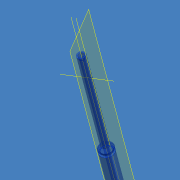
# Autodesk Inventor part: Halter02
Saved by Autodesk Inventor 2013 (Build 170138000, 138)
## iProperties
Created: 2006-08-08
Part Number: Halter02
Document SubType Name: Modeling
Designer: acad
Manufacturer: Standard
Standards Organization: Custom
Material: Allgemein
Density: 1 g/cm^3
Author: acad
Autodesk Inventor part; units mm, degrees
ref_plane "YZ Plane" through (0, 0, 0) normal (1, 0, 0) x (0, 1, 0)
ref_plane "XZ Plane" through (0, 0, 0) normal (0, 1, 0) x (-1, 0, 0)
ref_plane "XY Plane" through (0, 0, 0) normal (0, 0, 1) x (1, 0, 0)
sketch "Skizze1" plane through (0, 0, 0) normal (0, 0, 1) x (1, 0, 0)
  line L0 (-0.0085, 0) -> (-0.0085, 9)
  line L1 (-7.0085, 16) -> (-15.0085, 16)
  line L2 (-15.0085, 16) -> (-15.0085, 7)
  line L3 (-30.0085, 5.925) -> (-111.1085, 5.925)
  line L4 (-113.8085, 5.925) -> (-115.0085, 5.925)
  line L5 (-115.0085, 5.925) -> (-117.4335, 3.5)
  line L6 (-117.4335, 3.5) -> (-204.9135, 3.5)
  line L7 (-204.9135, 3.5) -> (-204.9135, 0)
  line L8 (-222.883, 3.2454) -> (-222.883, 3.2454)
  line L9 (-222.883, 3.2454) -> (-222.883, 3.2454)
  line L10 (-204.9135, 0) -> (-0.0085, 0)
  line L11 (-111.8085, 4.5) -> (-113.1085, 4.5)
  line L12 (-30.0085, 5.925) -> (-29.0085, 7)
  line L13 (-29.0085, 7) -> (-15.0085, 7)
  line L14 (-113.7085, 5.1) -> (-113.7085, 5.825)
  line L15 (-111.2085, 5.1) -> (-111.2085, 5.825)
  arc A0 (-113.7085, 5.1) -> (-113.1085, 4.5) centre (-113.1085, 5.1) ccw
  arc A1 (-111.8085, 4.5) -> (-111.2085, 5.1) centre (-111.8085, 5.1) ccw
  arc A2 (-111.1085, 5.925) -> (-111.2085, 5.825) centre (-111.1085, 5.825) ccw
  arc A3 (-113.7085, 5.825) -> (-113.8085, 5.925) centre (-113.8085, 5.825) ccw
  line L16 (-7.0085, 16) -> (-7.0085, 9)
  line L17 (-7.0085, 9) -> (-0.0085, 9)
  point P0 (-111.2085, 5.925)
  point P1 (-113.7085, 5.925)
  point P2 (-111.2085, 4.5)
  point P3 (-113.7085, 4.5)
  dimension "d19" = 14
  dimension "d20" = 15
  dimension "d21" = 7
  dimension "d22" = 5.925
  dimension "d23" = 4.5
  dimension "d24" = 3.5
  dimension "d26" = 47.07
  dimension "d27" = 45
  dimension "d33" = 2.5
  dimension "d34" = 1.3
  dimension "d35" = 87.48
  dimension "d44" = 0.6
  dimension "d45" = 0.1
  dimension "d127" = 16
  dimension "d128" = 8
  dimension "d129" = 7
  dimension "d130" = 9
  dimension "d152" = 189.905
  dimension "d153" = 174.905
  dimension "d154" = 111.2
  dimension "d156" = 81.2
  dimension "d157" = 2.425
  constraints: 36 end point, 10 parallel, 8 point on circle, 8 point on line, 8 tangent, 4 centre point, 4 perpendicular, 2 equal radius, 1 collinear, 1 vertical
  measures "d19" distance of L12.end L2.end
  measures "d20" horizontal distance of L2.end L3.start
  measures "d21" distance between parallel lines of L10 L13
  measures "d22" distance between parallel lines of L10 L3
  measures "d23" distance between parallel lines of L10 L11
  measures "d24" distance between parallel lines of L10 L6
  measures "d26" angle of L13 L12
  measures "d27" angle of L4 L5
  measures "d33" distance of point (-111.208, 4.5) point (-113.708, 4.5)
  measures "d34" distance of point (-113.708, 5.925) L4.end
  measures "d35" distance of L5.end L6.end
  measures "d44" radius of A0
  measures "d45" radius of A2
  measures "d127" distance between parallel lines of L10 L1
  measures "d128" distance of L1.start L1.end
  measures "d129" distance of L16.end L0.end
  measures "d130" distance of L0.start L0.end
  measures "d152" distance between parallel lines of L2 L7
  measures "d153" distance from line of L3.start L7
  measures "d154" distance between parallel lines of L0 L15
  measures "d156" distance from line of L3.start L15
  measures "d157" horizontal distance of L4.end L5.end
revolve "Drehung2" add sketch "Skizze1" angle 360 about axis through (-204.9135, 0, 0) along (1, 0, 0)
ref_plane "Arbeitsebene1" through (-161.1735, 3.5, 0) normal (0, 1, 0) x (-1, 0, 0)
sketch "Skizze3" plane through (-161.1735, 3.5, 0) normal (0, 1, 0) x (-1, 0, 0)
  line L0 (-43.74, 3.5) -> (-43.74, -3.5) projected
  line L1 (43.74, 3.5) -> (43.74, -3.5) projected
  line L2 (43.74, 3.5) -> (-43.74, 3.5) projected
  line L3 (43.74, -3.5) -> (-43.74, -3.5) projected
  line L4 (-222.6365, 0) -> (64.2305, 0) projected
  point P0 (21.74, 0)
  dimension "d158" = 65.48
  dimension "d166" = 22
  constraints: 1 point on line
  measures "d158" distance from line of L0 point (21.74, 0)
  measures "d166" distance from line of L1 point (21.74, 0)
hole "Bohrung1" at (-182.9135, 3.5, 0) direction (0, -1, 0) diameter 1.5 depth 3.5
hole "Bohrung2" at (-0.0085, 0, 0) direction (-1, 0, 0) diameter 4 depth 223
sketch "Skizze4" plane through (-15.0085, 0, 0) normal (-1, 0, 0) x (0, 0, 1)
  circle A0 centre (0, 0) radius 16 projected
  circle A1 centre (0, 0) radius 16 projected
  circle A2 centre (0, 0) radius 7 projected
  circle A3 centre (0, 0) radius 7 projected
  line L0 (0, -19.2) -> (0, 25.6) projected
  circle A4 centre (0, 0) radius 9 projected
  point P0 (-10, 0)
  point P1 (0, 11.7051)
  dimension "d132" = 90
  dimension "d148" = 10
  constraints: 1 point on line
  measures "d148" distance of A4.centre point (-10, 0)
hole "Bohrung3" at (-15.0085, 0, -10) direction (1, 0, 0) diameter 1.5 depth 8
sketch "Skizze17" plane through (-7.0085, 0, 0) normal (1, 0, 0) x (0, 0, -1)
  circle A0 centre (0, 0) radius 16 projected
  line L0 (0, -19.2) -> (0, 25.6) projected
  circle A1 centre (0, 0) radius 9 projected
  point P0 (0, 12.5)
  point P1 (0, -12.5)
  point P2 (0, 9)
  point P3 (0, 16)
  point P4 (0, -16)
  point P5 (0, -9)
  dimension "d135" = 7
  dimension "d136" = 3.5
  dimension "d137" = 3.5
  dimension "d145" = 12.5
  constraints: 6 point on line, 4 point on circle
  measures "d135" distance of A1.start A0.start
  measures "d136" distance of A1.start point (0, 12.5)
  measures "d137" distance of A1.end point (0, -12.5)
  measures "d145" distance of A0.centre point (0, 12.5)
hole "Bohrung10" at (-7.0085, -12.5, 0) at (-7.0085, 12.5, 0) direction (-1, 0, 0) diameter 1.567 depth 6 tip angle 118 thread size "M2x0.4" class "6H" standard "ANSI Metrisches M Profil"
sketch "Skizze19" plane through (-204.9135, 0, 0) normal (-1, 0, 0) x (0, 0, 1)
  circle A0 centre (0, 0) radius 2 projected
  constraints: 1 coincident
hole "Bohrung11" at (-204.9135, 0, 0) direction (1, 0, 0) diameter 5 depth 3
equation "\"d136\" = 0.5 * d135"
equation "\"d137\" = d136"
